Autodesk Fusion 360 part; units mm, degrees
(part 5 of 14)
  line L2140 (528.9162, 201.6125) -> (534.4154, 192.0875)
  line L2141 (534.4154, 192.0875) -> (545.4139, 192.0875)
  line L2142 (550.9132, 201.6125) -> (545.4139, 211.1375)
  line L2143 (545.4139, 192.0875) -> (550.9132, 201.6125)
  line L2144 (564.6614, 222.25) -> (553.6628, 222.25)
  line L2145 (553.6628, 222.25) -> (548.1636, 212.725)
  line L2146 (548.1636, 212.725) -> (553.6628, 203.2)
  line L2147 (553.6628, 203.2) -> (564.6614, 203.2)
  line L2148 (570.1606, 212.725) -> (564.6614, 222.25)
  line L2149 (564.6614, 203.2) -> (570.1606, 212.725)
  line L2150 (583.9088, 233.3625) -> (572.9102, 233.3625)
  line L2151 (572.9102, 233.3625) -> (567.411, 223.8375)
  line L2152 (567.411, 223.8375) -> (572.9102, 214.3125)
  line L2153 (572.9102, 214.3125) -> (583.9088, 214.3125)
  line L2154 (589.408, 223.8375) -> (583.9088, 233.3625)
  line L2155 (583.9088, 214.3125) -> (589.408, 223.8375)
  line L2156 (603.1562, 244.475) -> (592.1577, 244.475)
  line L2157 (592.1577, 244.475) -> (586.6584, 234.95)
  line L2158 (586.6584, 234.95) -> (592.1577, 225.425)
  line L2159 (592.1577, 225.425) -> (603.1562, 225.425)
  line L2160 (608.6554, 234.95) -> (603.1562, 244.475)
  line L2161 (603.1562, 225.425) -> (608.6554, 234.95)
  line L2162 (622.4036, 255.5875) -> (611.4051, 255.5875)
  line L2163 (611.4051, 255.5875) -> (605.9058, 246.0625)
  line L2164 (605.9058, 246.0625) -> (611.4051, 236.5375)
  line L2165 (611.4051, 236.5375) -> (622.4036, 236.5375)
  line L2166 (627.9029, 246.0625) -> (622.4036, 255.5875)
  line L2167 (622.4036, 236.5375) -> (627.9029, 246.0625)
  line L2168 (641.651, 266.7) -> (630.6525, 266.7)
  line L2169 (630.6525, 266.7) -> (625.1532, 257.175)
  line L2170 (625.1532, 257.175) -> (630.6525, 247.65)
  line L2171 (630.6525, 247.65) -> (641.651, 247.65)
  line L2172 (647.1503, 257.175) -> (641.651, 266.7)
  line L2173 (641.651, 247.65) -> (647.1503, 257.175)
  line L2174 (660.8984, 277.8125) -> (649.8999, 277.8125)
  line L2175 (649.8999, 277.8125) -> (644.4006, 268.2875)
  line L2176 (644.4006, 268.2875) -> (649.8999, 258.7625)
  line L2177 (649.8999, 258.7625) -> (660.8984, 258.7625)
  line L2178 (666.3977, 268.2875) -> (660.8984, 277.8125)
  line L2179 (660.8984, 258.7625) -> (666.3977, 268.2875)
  line L2180 (-493.9464, -366.7125) -> (-504.945, -366.7125)
  line L2181 (-504.945, -366.7125) -> (-510.4442, -376.2375)
  line L2182 (-510.4442, -376.2375) -> (-504.945, -385.7625)
  line L2183 (-504.945, -385.7625) -> (-493.9464, -385.7625)
  line L2184 (-488.4472, -376.2375) -> (-493.9464, -366.7125)
  line L2185 (-493.9464, -385.7625) -> (-488.4472, -376.2375)
  line L2186 (-474.699, -355.6) -> (-485.6976, -355.6)
  line L2187 (-485.6976, -355.6) -> (-491.1968, -365.125)
  line L2188 (-491.1968, -365.125) -> (-485.6976, -374.65)
  line L2189 (-485.6976, -374.65) -> (-474.699, -374.65)
  line L2190 (-469.1998, -365.125) -> (-474.699, -355.6)
  line L2191 (-474.699, -374.65) -> (-469.1998, -365.125)
  line L2192 (-455.4516, -344.4875) -> (-466.4501, -344.4875)
  line L2193 (-466.4501, -344.4875) -> (-471.9494, -354.0125)
  line L2194 (-471.9494, -354.0125) -> (-466.4501, -363.5375)
  line L2195 (-466.4501, -363.5375) -> (-455.4516, -363.5375)
  line L2196 (-449.9524, -354.0125) -> (-455.4516, -344.4875)
  line L2197 (-455.4516, -363.5375) -> (-449.9524, -354.0125)
  line L2198 (-436.2042, -333.375) -> (-447.2027, -333.375)
  line L2199 (-447.2027, -333.375) -> (-452.702, -342.9)
  line L2200 (-452.702, -342.9) -> (-447.2027, -352.425)
  line L2201 (-447.2027, -352.425) -> (-436.2042, -352.425)
  line L2202 (-430.7049, -342.9) -> (-436.2042, -333.375)
  line L2203 (-436.2042, -352.425) -> (-430.7049, -342.9)
  line L2204 (-416.9568, -322.2625) -> (-427.9553, -322.2625)
  line L2205 (-427.9553, -322.2625) -> (-433.4546, -331.7875)
  line L2206 (-433.4546, -331.7875) -> (-427.9553, -341.3125)
  line L2207 (-427.9553, -341.3125) -> (-416.9568, -341.3125)
  line L2208 (-411.4575, -331.7875) -> (-416.9568, -322.2625)
  line L2209 (-416.9568, -341.3125) -> (-411.4575, -331.7875)
  line L2210 (-397.7094, -311.15) -> (-408.7079, -311.15)
  line L2211 (-408.7079, -311.15) -> (-414.2072, -320.675)
  line L2212 (-414.2072, -320.675) -> (-408.7079, -330.2)
  line L2213 (-408.7079, -330.2) -> (-397.7094, -330.2)
  line L2214 (-392.2101, -320.675) -> (-397.7094, -311.15)
  line L2215 (-397.7094, -330.2) -> (-392.2101, -320.675)
  line L2216 (-378.462, -300.0375) -> (-389.4605, -300.0375)
  line L2217 (-389.4605, -300.0375) -> (-394.9597, -309.5625)
  line L2218 (-394.9597, -309.5625) -> (-389.4605, -319.0875)
  line L2219 (-389.4605, -319.0875) -> (-378.462, -319.0875)
  line L2220 (-372.9627, -309.5625) -> (-378.462, -300.0375)
  line L2221 (-378.462, -319.0875) -> (-372.9627, -309.5625)
  line L2222 (-359.2145, -288.925) -> (-370.2131, -288.925)
  line L2223 (-370.2131, -288.925) -> (-375.7123, -298.45)
  line L2224 (-375.7123, -298.45) -> (-370.2131, -307.975)
  line L2225 (-370.2131, -307.975) -> (-359.2145, -307.975)
  line L2226 (-353.7153, -298.45) -> (-359.2145, -288.925)
  line L2227 (-359.2145, -307.975) -> (-353.7153, -298.45)
  line L2228 (-339.9671, -277.8125) -> (-350.9657, -277.8125)
  line L2229 (-350.9657, -277.8125) -> (-356.4649, -287.3375)
  line L2230 (-356.4649, -287.3375) -> (-350.9657, -296.8625)
  line L2231 (-350.9657, -296.8625) -> (-339.9671, -296.8625)
  line L2232 (-334.4679, -287.3375) -> (-339.9671, -277.8125)
  line L2233 (-339.9671, -296.8625) -> (-334.4679, -287.3375)
  line L2234 (-320.7197, -266.7) -> (-331.7182, -266.7)
  line L2235 (-331.7182, -266.7) -> (-337.2175, -276.225)
  line L2236 (-337.2175, -276.225) -> (-331.7182, -285.75)
  line L2237 (-331.7182, -285.75) -> (-320.7197, -285.75)
  line L2238 (-315.2205, -276.225) -> (-320.7197, -266.7)
  line L2239 (-320.7197, -285.75) -> (-315.2205, -276.225)
  line L2240 (-301.4723, -255.5875) -> (-312.4708, -255.5875)
  line L2241 (-312.4708, -255.5875) -> (-317.9701, -265.1125)
  line L2242 (-317.9701, -265.1125) -> (-312.4708, -274.6375)
  line L2243 (-312.4708, -274.6375) -> (-301.4723, -274.6375)
  line L2244 (-295.973, -265.1125) -> (-301.4723, -255.5875)
  line L2245 (-301.4723, -274.6375) -> (-295.973, -265.1125)
  line L2246 (-282.2249, -244.475) -> (-293.2234, -244.475)
  line L2247 (-293.2234, -244.475) -> (-298.7227, -254)
  line L2248 (-298.7227, -254) -> (-293.2234, -263.525)
  line L2249 (-293.2234, -263.525) -> (-282.2249, -263.525)
  line L2250 (-276.7256, -254) -> (-282.2249, -244.475)
  line L2251 (-282.2249, -263.525) -> (-276.7256, -254)
  line L2252 (-262.9775, -233.3625) -> (-273.976, -233.3625)
  line L2253 (-273.976, -233.3625) -> (-279.4753, -242.8875)
  line L2254 (-279.4753, -242.8875) -> (-273.976, -252.4125)
  line L2255 (-273.976, -252.4125) -> (-262.9775, -252.4125)
  line L2256 (-257.4782, -242.8875) -> (-262.9775, -233.3625)
  line L2257 (-262.9775, -252.4125) -> (-257.4782, -242.8875)
  line L2258 (-243.7301, -222.25) -> (-254.7286, -222.25)
  line L2259 (-254.7286, -222.25) -> (-260.2278, -231.775)
  line L2260 (-260.2278, -231.775) -> (-254.7286, -241.3)
  line L2261 (-254.7286, -241.3) -> (-243.7301, -241.3)
  line L2262 (-238.2308, -231.775) -> (-243.7301, -222.25)
  line L2263 (-243.7301, -241.3) -> (-238.2308, -231.775)
  line L2264 (-224.4826, -211.1375) -> (-235.4812, -211.1375)
  line L2265 (-235.4812, -211.1375) -> (-240.9804, -220.6625)
  line L2266 (-240.9804, -220.6625) -> (-235.4812, -230.1875)
  line L2267 (-235.4812, -230.1875) -> (-224.4826, -230.1875)
  line L2268 (-218.9834, -220.6625) -> (-224.4826, -211.1375)
  line L2269 (-224.4826, -230.1875) -> (-218.9834, -220.6625)
  line L2270 (-205.2352, -200.025) -> (-216.2337, -200.025)
  line L2271 (-216.2337, -200.025) -> (-221.733, -209.55)
  line L2272 (-221.733, -209.55) -> (-216.2337, -219.075)
  line L2273 (-216.2337, -219.075) -> (-205.2352, -219.075)
  line L2274 (-199.736, -209.55) -> (-205.2352, -200.025)
  line L2275 (-205.2352, -219.075) -> (-199.736, -209.55)
  line L2276 (-185.9878, -188.9125) -> (-196.9863, -188.9125)
  line L2277 (-196.9863, -188.9125) -> (-202.4856, -198.4375)
  line L2278 (-202.4856, -198.4375) -> (-196.9863, -207.9625)
  line L2279 (-196.9863, -207.9625) -> (-185.9878, -207.9625)
  line L2280 (-180.4886, -198.4375) -> (-185.9878, -188.9125)
  line L2281 (-185.9878, -207.9625) -> (-180.4886, -198.4375)
  line L2282 (-166.7404, -177.8) -> (-177.7389, -177.8)
  line L2283 (-177.7389, -177.8) -> (-183.2382, -187.325)
  line L2284 (-183.2382, -187.325) -> (-177.7389, -196.85)
  line L2285 (-177.7389, -196.85) -> (-166.7404, -196.85)
  line L2286 (-161.2411, -187.325) -> (-166.7404, -177.8)
  line L2287 (-166.7404, -196.85) -> (-161.2411, -187.325)
  line L2288 (-147.493, -166.6875) -> (-158.4915, -166.6875)
  line L2289 (-158.4915, -166.6875) -> (-163.9908, -176.2125)
  line L2290 (-163.9908, -176.2125) -> (-158.4915, -185.7375)
  line L2291 (-158.4915, -185.7375) -> (-147.493, -185.7375)
  line L2292 (-141.9937, -176.2125) -> (-147.493, -166.6875)
  line L2293 (-147.493, -185.7375) -> (-141.9937, -176.2125)
  line L2294 (-128.2456, -155.575) -> (-139.2441, -155.575)
  line L2295 (-139.2441, -155.575) -> (-144.7434, -165.1)
  line L2296 (-144.7434, -165.1) -> (-139.2441, -174.625)
  line L2297 (-139.2441, -174.625) -> (-128.2456, -174.625)
  line L2298 (-122.7463, -165.1) -> (-128.2456, -155.575)
  line L2299 (-128.2456, -174.625) -> (-122.7463, -165.1)
  line L2300 (-108.9982, -144.4625) -> (-119.9967, -144.4625)
  line L2301 (-119.9967, -144.4625) -> (-125.4959, -153.9875)
  line L2302 (-125.4959, -153.9875) -> (-119.9967, -163.5125)
  line L2303 (-119.9967, -163.5125) -> (-108.9982, -163.5125)
  line L2304 (-103.4989, -153.9875) -> (-108.9982, -144.4625)
  line L2305 (-108.9982, -163.5125) -> (-103.4989, -153.9875)
  line L2306 (-89.7507, -133.35) -> (-100.7493, -133.35)
  line L2307 (-100.7493, -133.35) -> (-106.2485, -142.875)
  line L2308 (-106.2485, -142.875) -> (-100.7493, -152.4)
  line L2309 (-100.7493, -152.4) -> (-89.7507, -152.4)
  line L2310 (-84.2515, -142.875) -> (-89.7507, -133.35)
  line L2311 (-89.7507, -152.4) -> (-84.2515, -142.875)
  line L2312 (-70.5033, -122.2375) -> (-81.5018, -122.2375)
  line L2313 (-81.5018, -122.2375) -> (-87.0011, -131.7625)
  line L2314 (-87.0011, -131.7625) -> (-81.5018, -141.2875)
  line L2315 (-81.5018, -141.2875) -> (-70.5033, -141.2875)
  line L2316 (-65.0041, -131.7625) -> (-70.5033, -122.2375)
  line L2317 (-70.5033, -141.2875) -> (-65.0041, -131.7625)
  line L2318 (-51.2559, -111.125) -> (-62.2544, -111.125)
  line L2319 (-62.2544, -111.125) -> (-67.7537, -120.65)
  line L2320 (-67.7537, -120.65) -> (-62.2544, -130.175)
  line L2321 (-62.2544, -130.175) -> (-51.2559, -130.175)
  line L2322 (-45.7566, -120.65) -> (-51.2559, -111.125)
  line L2323 (-51.2559, -130.175) -> (-45.7566, -120.65)
  line L2324 (-32.0085, -100.0125) -> (-43.007, -100.0125)
  line L2325 (-43.007, -100.0125) -> (-48.5063, -109.5375)
  line L2326 (-48.5063, -109.5375) -> (-43.007, -119.0625)
  line L2327 (-43.007, -119.0625) -> (-32.0085, -119.0625)
  line L2328 (-26.5092, -109.5375) -> (-32.0085, -100.0125)
  line L2329 (-32.0085, -119.0625) -> (-26.5092, -109.5375)
  line L2330 (-12.7611, -88.9) -> (-23.7596, -88.9)
  line L2331 (-23.7596, -88.9) -> (-29.2589, -98.425)
  line L2332 (-29.2589, -98.425) -> (-23.7596, -107.95)
  line L2333 (-23.7596, -107.95) -> (-12.7611, -107.95)
  line L2334 (-7.2618, -98.425) -> (-12.7611, -88.9)
  line L2335 (-12.7611, -107.95) -> (-7.2618, -98.425)
  line L2336 (6.4863, -77.7875) -> (-4.5122, -77.7875)
  line L2337 (-4.5122, -77.7875) -> (-10.0114, -87.3125)
  line L2338 (-10.0114, -87.3125) -> (-4.5122, -96.8375)
  line L2339 (-4.5122, -96.8375) -> (6.4863, -96.8375)
  line L2340 (11.9856, -87.3125) -> (6.4863, -77.7875)
  line L2341 (6.4863, -96.8375) -> (11.9856, -87.3125)
  line L2342 (25.7337, -66.675) -> (14.7352, -66.675)
  line L2343 (14.7352, -66.675) -> (9.236, -76.2)
  line L2344 (9.236, -76.2) -> (14.7352, -85.725)
  line L2345 (14.7352, -85.725) -> (25.7337, -85.725)
  line L2346 (31.233, -76.2) -> (25.7337, -66.675)
  line L2347 (25.7337, -85.725) -> (31.233, -76.2)
  line L2348 (44.9812, -55.5625) -> (33.9826, -55.5625)
  line L2349 (33.9826, -55.5625) -> (28.4834, -65.0875)
  line L2350 (28.4834, -65.0875) -> (33.9826, -74.6125)
  line L2351 (33.9826, -74.6125) -> (44.9812, -74.6125)
  line L2352 (50.4804, -65.0875) -> (44.9812, -55.5625)
  line L2353 (44.9812, -74.6125) -> (50.4804, -65.0875)
  line L2354 (64.2286, -44.45) -> (53.2301, -44.45)
  line L2355 (53.2301, -44.45) -> (47.7308, -53.975)
  line L2356 (47.7308, -53.975) -> (53.2301, -63.5)
  line L2357 (53.2301, -63.5) -> (64.2286, -63.5)
  line L2358 (69.7278, -53.975) -> (64.2286, -44.45)
  line L2359 (64.2286, -63.5) -> (69.7278, -53.975)
  line L2360 (83.476, -33.3375) -> (72.4775, -33.3375)
  line L2361 (72.4775, -33.3375) -> (66.9782, -42.8625)
  line L2362 (66.9782, -42.8625) -> (72.4775, -52.3875)
  line L2363 (72.4775, -52.3875) -> (83.476, -52.3875)
  line L2364 (88.9753, -42.8625) -> (83.476, -33.3375)
  line L2365 (83.476, -52.3875) -> (88.9753, -42.8625)
  line L2366 (102.7234, -22.225) -> (91.7249, -22.225)
  line L2367 (91.7249, -22.225) -> (86.2256, -31.75)
  line L2368 (86.2256, -31.75) -> (91.7249, -41.275)
  line L2369 (91.7249, -41.275) -> (102.7234, -41.275)
  line L2370 (108.2227, -31.75) -> (102.7234, -22.225)
  line L2371 (102.7234, -41.275) -> (108.2227, -31.75)
  line L2372 (121.9708, -11.1125) -> (110.9723, -11.1125)
  line L2373 (110.9723, -11.1125) -> (105.473, -20.6375)
  line L2374 (105.473, -20.6375) -> (110.9723, -30.1625)
  line L2375 (110.9723, -30.1625) -> (121.9708, -30.1625)
  line L2376 (127.4701, -20.6375) -> (121.9708, -11.1125)
  line L2377 (121.9708, -30.1625) -> (127.4701, -20.6375)
  line L2378 (141.2182, 0) -> (130.2197, 0)
  line L2379 (130.2197, 0) -> (124.7205, -9.525)
  line L2380 (124.7205, -9.525) -> (130.2197, -19.05)
  line L2381 (130.2197, -19.05) -> (141.2182, -19.05)
  line L2382 (146.7175, -9.525) -> (141.2182, 0)
  line L2383 (141.2182, -19.05) -> (146.7175, -9.525)
  line L2384 (160.4657, 11.1125) -> (149.4671, 11.1125)
  line L2385 (149.4671, 11.1125) -> (143.9679, 1.5875)
  line L2386 (143.9679, 1.5875) -> (149.4671, -7.9375)
  line L2387 (149.4671, -7.9375) -> (160.4657, -7.9375)
  line L2388 (165.9649, 1.5875) -> (160.4657, 11.1125)
  line L2389 (160.4657, -7.9375) -> (165.9649, 1.5875)
  line L2390 (179.7131, 22.225) -> (168.7145, 22.225)
  line L2391 (168.7145, 22.225) -> (163.2153, 12.7)
  line L2392 (163.2153, 12.7) -> (168.7145, 3.175)
  line L2393 (168.7145, 3.175) -> (179.7131, 3.175)
  line L2394 (185.2123, 12.7) -> (179.7131, 22.225)
  line L2395 (179.7131, 3.175) -> (185.2123, 12.7)
  line L2396 (198.9605, 33.3375) -> (187.962, 33.3375)
  line L2397 (187.962, 33.3375) -> (182.4627, 23.8125)
  line L2398 (182.4627, 23.8125) -> (187.962, 14.2875)
  line L2399 (187.962, 14.2875) -> (198.9605, 14.2875)
  line L2400 (204.4597, 23.8125) -> (198.9605, 33.3375)
  line L2401 (198.9605, 14.2875) -> (204.4597, 23.8125)
  line L2402 (218.2079, 44.45) -> (207.2094, 44.45)
  line L2403 (207.2094, 44.45) -> (201.7101, 34.925)
  line L2404 (201.7101, 34.925) -> (207.2094, 25.4)
  line L2405 (207.2094, 25.4) -> (218.2079, 25.4)
  line L2406 (223.7072, 34.925) -> (218.2079, 44.45)
  line L2407 (218.2079, 25.4) -> (223.7072, 34.925)
  line L2408 (237.4553, 55.5625) -> (226.4568, 55.5625)
  line L2409 (226.4568, 55.5625) -> (220.9575, 46.0375)
  line L2410 (220.9575, 46.0375) -> (226.4568, 36.5125)
  line L2411 (226.4568, 36.5125) -> (237.4553, 36.5125)
  line L2412 (242.9546, 46.0375) -> (237.4553, 55.5625)
  line L2413 (237.4553, 36.5125) -> (242.9546, 46.0375)
  line L2414 (256.7027, 66.675) -> (245.7042, 66.675)
  line L2415 (245.7042, 66.675) -> (240.2049, 57.15)
  line L2416 (240.2049, 57.15) -> (245.7042, 47.625)
  line L2417 (245.7042, 47.625) -> (256.7027, 47.625)
  line L2418 (262.202, 57.15) -> (256.7027, 66.675)
  line L2419 (256.7027, 47.625) -> (262.202, 57.15)
  line L2420 (275.9501, 77.7875) -> (264.9516, 77.7875)
  line L2421 (264.9516, 77.7875) -> (259.4524, 68.2625)
  line L2422 (259.4524, 68.2625) -> (264.9516, 58.7375)
  line L2423 (264.9516, 58.7375) -> (275.9501, 58.7375)
  line L2424 (281.4494, 68.2625) -> (275.9501, 77.7875)
  line L2425 (275.9501, 58.7375) -> (281.4494, 68.2625)
  line L2426 (295.1976, 88.9) -> (284.199, 88.9)
  line L2427 (284.199, 88.9) -> (278.6998, 79.375)
  line L2428 (278.6998, 79.375) -> (284.199, 69.85)
  line L2429 (284.199, 69.85) -> (295.1976, 69.85)
  line L2430 (300.6968, 79.375) -> (295.1976, 88.9)
  line L2431 (295.1976, 69.85) -> (300.6968, 79.375)
  line L2432 (314.445, 100.0125) -> (303.4464, 100.0125)
  line L2433 (303.4464, 100.0125) -> (297.9472, 90.4875)
  line L2434 (297.9472, 90.4875) -> (303.4464, 80.9625)
  line L2435 (303.4464, 80.9625) -> (314.445, 80.9625)
  line L2436 (319.9442, 90.4875) -> (314.445, 100.0125)
  line L2437 (314.445, 80.9625) -> (319.9442, 90.4875)
  line L2438 (333.6924, 111.125) -> (322.6939, 111.125)
  line L2439 (322.6939, 111.125) -> (317.1946, 101.6)
  line L2440 (317.1946, 101.6) -> (322.6939, 92.075)
  line L2441 (322.6939, 92.075) -> (333.6924, 92.075)
  line L2442 (339.1916, 101.6) -> (333.6924, 111.125)
  line L2443 (333.6924, 92.075) -> (339.1916, 101.6)
  line L2444 (352.9398, 122.2375) -> (341.9413, 122.2375)
  line L2445 (341.9413, 122.2375) -> (336.442, 112.7125)
  line L2446 (336.442, 112.7125) -> (341.9413, 103.1875)
  line L2447 (341.9413, 103.1875) -> (352.9398, 103.1875)
  line L2448 (358.4391, 112.7125) -> (352.9398, 122.2375)
  line L2449 (352.9398, 103.1875) -> (358.4391, 112.7125)
  line L2450 (372.1872, 133.35) -> (361.1887, 133.35)
  line L2451 (361.1887, 133.35) -> (355.6894, 123.825)
  line L2452 (355.6894, 123.825) -> (361.1887, 114.3)
  line L2453 (361.1887, 114.3) -> (372.1872, 114.3)
  line L2454 (377.6865, 123.825) -> (372.1872, 133.35)
  line L2455 (372.1872, 114.3) -> (377.6865, 123.825)
  line L2456 (391.4346, 144.4625) -> (380.4361, 144.4625)
  line L2457 (380.4361, 144.4625) -> (374.9368, 134.9375)
  line L2458 (374.9368, 134.9375) -> (380.4361, 125.4125)
  line L2459 (380.4361, 125.4125) -> (391.4346, 125.4125)
  line L2460 (396.9339, 134.9375) -> (391.4346, 144.4625)
  line L2461 (391.4346, 125.4125) -> (396.9339, 134.9375)
  line L2462 (410.682, 155.575) -> (399.6835, 155.575)
  line L2463 (399.6835, 155.575) -> (394.1843, 146.05)
  line L2464 (394.1843, 146.05) -> (399.6835, 136.525)
  line L2465 (399.6835, 136.525) -> (410.682, 136.525)
  line L2466 (416.1813, 146.05) -> (410.682, 155.575)
  line L2467 (410.682, 136.525) -> (416.1813, 146.05)
  line L2468 (429.9295, 166.6875) -> (418.9309, 166.6875)
  line L2469 (418.9309, 166.6875) -> (413.4317, 157.1625)
  line L2470 (413.4317, 157.1625) -> (418.9309, 147.6375)
  line L2471 (418.9309, 147.6375) -> (429.9295, 147.6375)
  line L2472 (435.4287, 157.1625) -> (429.9295, 166.6875)
  line L2473 (429.9295, 147.6375) -> (435.4287, 157.1625)
  line L2474 (449.1769, 177.8) -> (438.1783, 177.8)
  line L2475 (438.1783, 177.8) -> (432.6791, 168.275)
  line L2476 (432.6791, 168.275) -> (438.1783, 158.75)
  line L2477 (438.1783, 158.75) -> (449.1769, 158.75)
  line L2478 (454.6761, 168.275) -> (449.1769, 177.8)
  line L2479 (449.1769, 158.75) -> (454.6761, 168.275)
  line L2480 (468.4243, 188.9125) -> (457.4258, 188.9125)
  line L2481 (457.4258, 188.9125) -> (451.9265, 179.3875)
  line L2482 (451.9265, 179.3875) -> (457.4258, 169.8625)
  line L2483 (457.4258, 169.8625) -> (468.4243, 169.8625)
  line L2484 (473.9235, 179.3875) -> (468.4243, 188.9125)
  line L2485 (468.4243, 169.8625) -> (473.9235, 179.3875)
  line L2486 (487.6717, 200.025) -> (476.6732, 200.025)
  line L2487 (476.6732, 200.025) -> (471.1739, 190.5)
  line L2488 (471.1739, 190.5) -> (476.6732, 180.975)
  line L2489 (476.6732, 180.975) -> (487.6717, 180.975)
  line L2490 (493.171, 190.5) -> (487.6717, 200.025)
  line L2491 (487.6717, 180.975) -> (493.171, 190.5)
  line L2492 (506.9191, 211.1375) -> (495.9206, 211.1375)
  line L2493 (495.9206, 211.1375) -> (490.4213, 201.6125)
  line L2494 (490.4213, 201.6125) -> (495.9206, 192.0875)
  line L2495 (495.9206, 192.0875) -> (506.9191, 192.0875)
  line L2496 (512.4184, 201.6125) -> (506.9191, 211.1375)
  line L2497 (506.9191, 192.0875) -> (512.4184, 201.6125)
  line L2498 (526.1665, 222.25) -> (515.168, 222.25)
  line L2499 (515.168, 222.25) -> (509.6687, 212.725)
  line L2500 (509.6687, 212.725) -> (515.168, 203.2)
  line L2501 (515.168, 203.2) -> (526.1665, 203.2)
  line L2502 (531.6658, 212.725) -> (526.1665, 222.25)
  line L2503 (526.1665, 203.2) -> (531.6658, 212.725)
  line L2504 (545.4139, 233.3625) -> (534.4154, 233.3625)
  line L2505 (534.4154, 233.3625) -> (528.9162, 223.8375)
  line L2506 (528.9162, 223.8375) -> (534.4154, 214.3125)
  line L2507 (534.4154, 214.3125) -> (545.4139, 214.3125)
  line L2508 (550.9132, 223.8375) -> (545.4139, 233.3625)
  line L2509 (545.4139, 214.3125) -> (550.9132, 223.8375)
  line L2510 (564.6614, 244.475) -> (553.6628, 244.475)
  line L2511 (553.6628, 244.475) -> (548.1636, 234.95)
  line L2512 (548.1636, 234.95) -> (553.6628, 225.425)
  line L2513 (553.6628, 225.425) -> (564.6614, 225.425)
  line L2514 (570.1606, 234.95) -> (564.6614, 244.475)
  line L2515 (564.6614, 225.425) -> (570.1606, 234.95)
  line L2516 (583.9088, 255.5875) -> (572.9102, 255.5875)
  line L2517 (572.9102, 255.5875) -> (567.411, 246.0625)
  line L2518 (567.411, 246.0625) -> (572.9102, 236.5375)
  line L2519 (572.9102, 236.5375) -> (583.9088, 236.5375)
  line L2520 (589.408, 246.0625) -> (583.9088, 255.5875)
  line L2521 (583.9088, 236.5375) -> (589.408, 246.0625)
  line L2522 (603.1562, 266.7) -> (592.1577, 266.7)
  line L2523 (592.1577, 266.7) -> (586.6584, 257.175)
  line L2524 (586.6584, 257.175) -> (592.1577, 247.65)
  line L2525 (592.1577, 247.65) -> (603.1562, 247.65)
  line L2526 (608.6554, 257.175) -> (603.1562, 266.7)
  line L2527 (603.1562, 247.65) -> (608.6554, 257.175)
  line L2528 (622.4036, 277.8125) -> (611.4051, 277.8125)
  line L2529 (611.4051, 277.8125) -> (605.9058, 268.2875)
  line L2530 (605.9058, 268.2875) -> (611.4051, 258.7625)
  line L2531 (611.4051, 258.7625) -> (622.4036, 258.7625)
  line L2532 (627.9029, 268.2875) -> (622.4036, 277.8125)
  line L2533 (622.4036, 258.7625) -> (627.9029, 268.2875)
  line L2534 (641.651, 288.925) -> (630.6525, 288.925)
  line L2535 (630.6525, 288.925) -> (625.1532, 279.4)
  line L2536 (625.1532, 279.4) -> (630.6525, 269.875)
  line L2537 (630.6525, 269.875) -> (641.651, 269.875)
  line L2538 (647.1503, 279.4) -> (641.651, 288.925)
  line L2539 (641.651, 269.875) -> (647.1503, 279.4)
  line L2540 (-513.1939, -355.6) -> (-524.1924, -355.6)
  line L2541 (-524.1924, -355.6) -> (-529.6916, -365.125)
  line L2542 (-529.6916, -365.125) -> (-524.1924, -374.65)
  line L2543 (-524.1924, -374.65) -> (-513.1939, -374.65)
  line L2544 (-507.6946, -365.125) -> (-513.1939, -355.6)
  line L2545 (-513.1939, -374.65) -> (-507.6946, -365.125)
  line L2546 (-493.9464, -344.4875) -> (-504.945, -344.4875)
  line L2547 (-504.945, -344.4875) -> (-510.4442, -354.0125)
  line L2548 (-510.4442, -354.0125) -> (-504.945, -363.5375)
  line L2549 (-504.945, -363.5375) -> (-493.9464, -363.5375)
  line L2550 (-488.4472, -354.0125) -> (-493.9464, -344.4875)
  line L2551 (-493.9464, -363.5375) -> (-488.4472, -354.0125)
  line L2552 (-474.699, -333.375) -> (-485.6976, -333.375)
  line L2553 (-485.6976, -333.375) -> (-491.1968, -342.9)
  line L2554 (-491.1968, -342.9) -> (-485.6976, -352.425)
  line L2555 (-485.6976, -352.425) -> (-474.699, -352.425)
  line L2556 (-469.1998, -342.9) -> (-474.699, -333.375)
  line L2557 (-474.699, -352.425) -> (-469.1998, -342.9)
  line L2558 (-455.4516, -322.2625) -> (-466.4501, -322.2625)
  line L2559 (-466.4501, -322.2625) -> (-471.9494, -331.7875)
  line L2560 (-471.9494, -331.7875) -> (-466.4501, -341.3125)
  line L2561 (-466.4501, -341.3125) -> (-455.4516, -341.3125)
  line L2562 (-449.9524, -331.7875) -> (-455.4516, -322.2625)
  line L2563 (-455.4516, -341.3125) -> (-449.9524, -331.7875)
  line L2564 (-436.2042, -311.15) -> (-447.2027, -311.15)
  line L2565 (-447.2027, -311.15) -> (-452.702, -320.675)
  line L2566 (-452.702, -320.675) -> (-447.2027, -330.2)
  line L2567 (-447.2027, -330.2) -> (-436.2042, -330.2)
  line L2568 (-430.7049, -320.675) -> (-436.2042, -311.15)
  line L2569 (-436.2042, -330.2) -> (-430.7049, -320.675)
  line L2570 (-416.9568, -300.0375) -> (-427.9553, -300.0375)
  line L2571 (-427.9553, -300.0375) -> (-433.4546, -309.5625)
  line L2572 (-433.4546, -309.5625) -> (-427.9553, -319.0875)
  line L2573 (-427.9553, -319.0875) -> (-416.9568, -319.0875)
  line L2574 (-411.4575, -309.5625) -> (-416.9568, -300.0375)
  line L2575 (-416.9568, -319.0875) -> (-411.4575, -309.5625)
  line L2576 (-397.7094, -288.925) -> (-408.7079, -288.925)
  line L2577 (-408.7079, -288.925) -> (-414.2072, -298.45)
  line L2578 (-414.2072, -298.45) -> (-408.7079, -307.975)
  line L2579 (-408.7079, -307.975) -> (-397.7094, -307.975)
  line L2580 (-392.2101, -298.45) -> (-397.7094, -288.925)
  line L2581 (-397.7094, -307.975) -> (-392.2101, -298.45)
  line L2582 (-378.462, -277.8125) -> (-389.4605, -277.8125)
  line L2583 (-389.4605, -277.8125) -> (-394.9597, -287.3375)
  line L2584 (-394.9597, -287.3375) -> (-389.4605, -296.8625)
  line L2585 (-389.4605, -296.8625) -> (-378.462, -296.8625)
  line L2586 (-372.9627, -287.3375) -> (-378.462, -277.8125)
  line L2587 (-378.462, -296.8625) -> (-372.9627, -287.3375)
  line L2588 (-359.2145, -266.7) -> (-370.2131, -266.7)
  line L2589 (-370.2131, -266.7) -> (-375.7123, -276.225)
  line L2590 (-375.7123, -276.225) -> (-370.2131, -285.75)
  line L2591 (-370.2131, -285.75) -> (-359.2145, -285.75)
  line L2592 (-353.7153, -276.225) -> (-359.2145, -266.7)
  line L2593 (-359.2145, -285.75) -> (-353.7153, -276.225)
  line L2594 (-339.9671, -255.5875) -> (-350.9657, -255.5875)
  line L2595 (-350.9657, -255.5875) -> (-356.4649, -265.1125)
  line L2596 (-356.4649, -265.1125) -> (-350.9657, -274.6375)
  line L2597 (-350.9657, -274.6375) -> (-339.9671, -274.6375)
  line L2598 (-334.4679, -265.1125) -> (-339.9671, -255.5875)
  line L2599 (-339.9671, -274.6375) -> (-334.4679, -265.1125)
  line L2600 (-320.7197, -244.475) -> (-331.7182, -244.475)
  line L2601 (-331.7182, -244.475) -> (-337.2175, -254)
  line L2602 (-337.2175, -254) -> (-331.7182, -263.525)
  line L2603 (-331.7182, -263.525) -> (-320.7197, -263.525)
  line L2604 (-315.2205, -254) -> (-320.7197, -244.475)
  line L2605 (-320.7197, -263.525) -> (-315.2205, -254)
  line L2606 (-301.4723, -233.3625) -> (-312.4708, -233.3625)
  line L2607 (-312.4708, -233.3625) -> (-317.9701, -242.8875)
  line L2608 (-317.9701, -242.8875) -> (-312.4708, -252.4125)
  line L2609 (-312.4708, -252.4125) -> (-301.4723, -252.4125)
  line L2610 (-295.973, -242.8875) -> (-301.4723, -233.3625)
  line L2611 (-301.4723, -252.4125) -> (-295.973, -242.8875)
  line L2612 (-282.2249, -222.25) -> (-293.2234, -222.25)
  line L2613 (-293.2234, -222.25) -> (-298.7227, -231.775)
  line L2614 (-298.7227, -231.775) -> (-293.2234, -241.3)
  line L2615 (-293.2234, -241.3) -> (-282.2249, -241.3)
  line L2616 (-276.7256, -231.775) -> (-282.2249, -222.25)
  line L2617 (-282.2249, -241.3) -> (-276.7256, -231.775)
  line L2618 (-262.9775, -211.1375) -> (-273.976, -211.1375)
  line L2619 (-273.976, -211.1375) -> (-279.4753, -220.6625)
  line L2620 (-279.4753, -220.6625) -> (-273.976, -230.1875)
  line L2621 (-273.976, -230.1875) -> (-262.9775, -230.1875)
  line L2622 (-257.4782, -220.6625) -> (-262.9775, -211.1375)
  line L2623 (-262.9775, -230.1875) -> (-257.4782, -220.6625)
  line L2624 (-243.7301, -200.025) -> (-254.7286, -200.025)
  line L2625 (-254.7286, -200.025) -> (-260.2278, -209.55)
  line L2626 (-260.2278, -209.55) -> (-254.7286, -219.075)
  line L2627 (-254.7286, -219.075) -> (-243.7301, -219.075)
  line L2628 (-238.2308, -209.55) -> (-243.7301, -200.025)
  line L2629 (-243.7301, -219.075) -> (-238.2308, -209.55)
  line L2630 (-224.4826, -188.9125) -> (-235.4812, -188.9125)
  line L2631 (-235.4812, -188.9125) -> (-240.9804, -198.4375)
  line L2632 (-240.9804, -198.4375) -> (-235.4812, -207.9625)
  line L2633 (-235.4812, -207.9625) -> (-224.4826, -207.9625)
  line L2634 (-218.9834, -198.4375) -> (-224.4826, -188.9125)
  line L2635 (-224.4826, -207.9625) -> (-218.9834, -198.4375)
  line L2636 (-205.2352, -177.8) -> (-216.2337, -177.8)
  line L2637 (-216.2337, -177.8) -> (-221.733, -187.325)
  line L2638 (-221.733, -187.325) -> (-216.2337, -196.85)
  line L2639 (-216.2337, -196.85) -> (-205.2352, -196.85)
  line L2640 (-199.736, -187.325) -> (-205.2352, -177.8)
  line L2641 (-205.2352, -196.85) -> (-199.736, -187.325)
  line L2642 (-185.9878, -166.6875) -> (-196.9863, -166.6875)
  line L2643 (-196.9863, -166.6875) -> (-202.4856, -176.2125)
  line L2644 (-202.4856, -176.2125) -> (-196.9863, -185.7375)
  line L2645 (-196.9863, -185.7375) -> (-185.9878, -185.7375)
  line L2646 (-180.4886, -176.2125) -> (-185.9878, -166.6875)
  line L2647 (-185.9878, -185.7375) -> (-180.4886, -176.2125)
  line L2648 (-166.7404, -155.575) -> (-177.7389, -155.575)
  line L2649 (-177.7389, -155.575) -> (-183.2382, -165.1)
  line L2650 (-183.2382, -165.1) -> (-177.7389, -174.625)
  line L2651 (-177.7389, -174.625) -> (-166.7404, -174.625)
  line L2652 (-161.2411, -165.1) -> (-166.7404, -155.575)
  line L2653 (-166.7404, -174.625) -> (-161.2411, -165.1)
  line L2654 (-147.493, -144.4625) -> (-158.4915, -144.4625)
  line L2655 (-158.4915, -144.4625) -> (-163.9908, -153.9875)
  line L2656 (-163.9908, -153.9875) -> (-158.4915, -163.5125)
  line L2657 (-158.4915, -163.5125) -> (-147.493, -163.5125)
  line L2658 (-141.9937, -153.9875) -> (-147.493, -144.4625)
  line L2659 (-147.493, -163.5125) -> (-141.9937, -153.9875)
  line L2660 (-128.2456, -133.35) -> (-139.2441, -133.35)
  line L2661 (-139.2441, -133.35) -> (-144.7434, -142.875)
  line L2662 (-144.7434, -142.875) -> (-139.2441, -152.4)
  line L2663 (-139.2441, -152.4) -> (-128.2456, -152.4)
  line L2664 (-122.7463, -142.875) -> (-128.2456, -133.35)
  line L2665 (-128.2456, -152.4) -> (-122.7463, -142.875)
  line L2666 (-108.9982, -122.2375) -> (-119.9967, -122.2375)
  line L2667 (-119.9967, -122.2375) -> (-125.4959, -131.7625)
  line L2668 (-125.4959, -131.7625) -> (-119.9967, -141.2875)
  line L2669 (-119.9967, -141.2875) -> (-108.9982, -141.2875)
  line L2670 (-103.4989, -131.7625) -> (-108.9982, -122.2375)
  line L2671 (-108.9982, -141.2875) -> (-103.4989, -131.7625)
  line L2672 (-89.7507, -111.125) -> (-100.7493, -111.125)
  line L2673 (-100.7493, -111.125) -> (-106.2485, -120.65)
  line L2674 (-106.2485, -120.65) -> (-100.7493, -130.175)
  line L2675 (-100.7493, -130.175) -> (-89.7507, -130.175)
  line L2676 (-84.2515, -120.65) -> (-89.7507, -111.125)
  line L2677 (-89.7507, -130.175) -> (-84.2515, -120.65)
  line L2678 (-70.5033, -100.0125) -> (-81.5018, -100.0125)
  line L2679 (-81.5018, -100.0125) -> (-87.0011, -109.5375)
  line L2680 (-87.0011, -109.5375) -> (-81.5018, -119.0625)
  line L2681 (-81.5018, -119.0625) -> (-70.5033, -119.0625)
  line L2682 (-65.0041, -109.5375) -> (-70.5033, -100.0125)
  line L2683 (-70.5033, -119.0625) -> (-65.0041, -109.5375)
  line L2684 (-51.2559, -88.9) -> (-62.2544, -88.9)
  line L2685 (-62.2544, -88.9) -> (-67.7537, -98.425)
  line L2686 (-67.7537, -98.425) -> (-62.2544, -107.95)
  line L2687 (-62.2544, -107.95) -> (-51.2559, -107.95)
  line L2688 (-45.7566, -98.425) -> (-51.2559, -88.9)
  line L2689 (-51.2559, -107.95) -> (-45.7566, -98.425)
  line L2690 (-32.0085, -77.7875) -> (-43.007, -77.7875)
  line L2691 (-43.007, -77.7875) -> (-48.5063, -87.3125)
  line L2692 (-48.5063, -87.3125) -> (-43.007, -96.8375)
  line L2693 (-43.007, -96.8375) -> (-32.0085, -96.8375)
  line L2694 (-26.5092, -87.3125) -> (-32.0085, -77.7875)
  line L2695 (-32.0085, -96.8375) -> (-26.5092, -87.3125)
  line L2696 (-12.7611, -66.675) -> (-23.7596, -66.675)
  line L2697 (-23.7596, -66.675) -> (-29.2589, -76.2)
  line L2698 (-29.2589, -76.2) -> (-23.7596, -85.725)
  line L2699 (-23.7596, -85.725) -> (-12.7611, -85.725)
  line L2700 (-7.2618, -76.2) -> (-12.7611, -66.675)
  line L2701 (-12.7611, -85.725) -> (-7.2618, -76.2)
  line L2702 (6.4863, -55.5625) -> (-4.5122, -55.5625)
  line L2703 (-4.5122, -55.5625) -> (-10.0114, -65.0875)
  line L2704 (-10.0114, -65.0875) -> (-4.5122, -74.6125)
  line L2705 (-4.5122, -74.6125) -> (6.4863, -74.6125)
  line L2706 (11.9856, -65.0875) -> (6.4863, -55.5625)
  line L2707 (6.4863, -74.6125) -> (11.9856, -65.0875)
  line L2708 (25.7337, -44.45) -> (14.7352, -44.45)
  line L2709 (14.7352, -44.45) -> (9.236, -53.975)
  line L2710 (9.236, -53.975) -> (14.7352, -63.5)
  line L2711 (14.7352, -63.5) -> (25.7337, -63.5)
  line L2712 (31.233, -53.975) -> (25.7337, -44.45)
  line L2713 (25.7337, -63.5) -> (31.233, -53.975)
  line L2714 (44.9812, -33.3375) -> (33.9826, -33.3375)
  line L2715 (33.9826, -33.3375) -> (28.4834, -42.8625)
  line L2716 (28.4834, -42.8625) -> (33.9826, -52.3875)
  line L2717 (33.9826, -52.3875) -> (44.9812, -52.3875)
  line L2718 (50.4804, -42.8625) -> (44.9812, -33.3375)
  line L2719 (44.9812, -52.3875) -> (50.4804, -42.8625)
  line L2720 (64.2286, -22.225) -> (53.2301, -22.225)
  line L2721 (53.2301, -22.225) -> (47.7308, -31.75)
  line L2722 (47.7308, -31.75) -> (53.2301, -41.275)
  line L2723 (53.2301, -41.275) -> (64.2286, -41.275)
  line L2724 (69.7278, -31.75) -> (64.2286, -22.225)
  line L2725 (64.2286, -41.275) -> (69.7278, -31.75)
  line L2726 (83.476, -11.1125) -> (72.4775, -11.1125)
  line L2727 (72.4775, -11.1125) -> (66.9782, -20.6375)
  line L2728 (66.9782, -20.6375) -> (72.4775, -30.1625)
  line L2729 (72.4775, -30.1625) -> (83.476, -30.1625)
  line L2730 (88.9753, -20.6375) -> (83.476, -11.1125)
  line L2731 (83.476, -30.1625) -> (88.9753, -20.6375)
  line L2732 (102.7234, 0) -> (91.7249, 0)
  line L2733 (91.7249, 0) -> (86.2256, -9.525)
  line L2734 (86.2256, -9.525) -> (91.7249, -19.05)
  line L2735 (91.7249, -19.05) -> (102.7234, -19.05)
  line L2736 (108.2227, -9.525) -> (102.7234, 0)
  line L2737 (102.7234, -19.05) -> (108.2227, -9.525)
  line L2738 (121.9708, 11.1125) -> (110.9723, 11.1125)
  line L2739 (110.9723, 11.1125) -> (105.473, 1.5875)
  line L2740 (105.473, 1.5875) -> (110.9723, -7.9375)
  line L2741 (110.9723, -7.9375) -> (121.9708, -7.9375)
  line L2742 (127.4701, 1.5875) -> (121.9708, 11.1125)
  line L2743 (121.9708, -7.9375) -> (127.4701, 1.5875)
  line L2744 (141.2182, 22.225) -> (130.2197, 22.225)
  line L2745 (130.2197, 22.225) -> (124.7205, 12.7)
  line L2746 (124.7205, 12.7) -> (130.2197, 3.175)
  line L2747 (130.2197, 3.175) -> (141.2182, 3.175)
  line L2748 (146.7175, 12.7) -> (141.2182, 22.225)
  line L2749 (141.2182, 3.175) -> (146.7175, 12.7)
  line L2750 (160.4657, 33.3375) -> (149.4671, 33.3375)
  line L2751 (149.4671, 33.3375) -> (143.9679, 23.8125)
  line L2752 (143.9679, 23.8125) -> (149.4671, 14.2875)
  line L2753 (149.4671, 14.2875) -> (160.4657, 14.2875)
  line L2754 (165.9649, 23.8125) -> (160.4657, 33.3375)
  line L2755 (160.4657, 14.2875) -> (165.9649, 23.8125)
  line L2756 (179.7131, 44.45) -> (168.7145, 44.45)
  line L2757 (168.7145, 44.45) -> (163.2153, 34.925)
  line L2758 (163.2153, 34.925) -> (168.7145, 25.4)
  line L2759 (168.7145, 25.4) -> (179.7131, 25.4)
  line L2760 (185.2123, 34.925) -> (179.7131, 44.45)
  line L2761 (179.7131, 25.4) -> (185.2123, 34.925)
  line L2762 (198.9605, 55.5625) -> (187.962, 55.5625)
  line L2763 (187.962, 55.5625) -> (182.4627, 46.0375)
  line L2764 (182.4627, 46.0375) -> (187.962, 36.5125)
  line L2765 (187.962, 36.5125) -> (198.9605, 36.5125)
  line L2766 (204.4597, 46.0375) -> (198.9605, 55.5625)
  line L2767 (198.9605, 36.5125) -> (204.4597, 46.0375)
  line L2768 (218.2079, 66.675) -> (207.2094, 66.675)
  line L2769 (207.2094, 66.675) -> (201.7101, 57.15)
  line L2770 (201.7101, 57.15) -> (207.2094, 47.625)
  line L2771 (207.2094, 47.625) -> (218.2079, 47.625)
  line L2772 (223.7072, 57.15) -> (218.2079, 66.675)
  line L2773 (218.2079, 47.625) -> (223.7072, 57.15)
  line L2774 (237.4553, 77.7875) -> (226.4568, 77.7875)
  line L2775 (226.4568, 77.7875) -> (220.9575, 68.2625)
  line L2776 (220.9575, 68.2625) -> (226.4568, 58.7375)
  line L2777 (226.4568, 58.7375) -> (237.4553, 58.7375)
  line L2778 (242.9546, 68.2625) -> (237.4553, 77.7875)
  line L2779 (237.4553, 58.7375) -> (242.9546, 68.2625)
  line L2780 (256.7027, 88.9) -> (245.7042, 88.9)
  line L2781 (245.7042, 88.9) -> (240.2049, 79.375)
  line L2782 (240.2049, 79.375) -> (245.7042, 69.85)
  line L2783 (245.7042, 69.85) -> (256.7027, 69.85)
  line L2784 (262.202, 79.375) -> (256.7027, 88.9)
  line L2785 (256.7027, 69.85) -> (262.202, 79.375)
  line L2786 (275.9501, 100.0125) -> (264.9516, 100.0125)
  line L2787 (264.9516, 100.0125) -> (259.4524, 90.4875)
  line L2788 (259.4524, 90.4875) -> (264.9516, 80.9625)
  line L2789 (264.9516, 80.9625) -> (275.9501, 80.9625)
  line L2790 (281.4494, 90.4875) -> (275.9501, 100.0125)
  line L2791 (275.9501, 80.9625) -> (281.4494, 90.4875)
  line L2792 (295.1976, 111.125) -> (284.199, 111.125)
  line L2793 (284.199, 111.125) -> (278.6998, 101.6)
  line L2794 (278.6998, 101.6) -> (284.199, 92.075)
  line L2795 (284.199, 92.075) -> (295.1976, 92.075)
  line L2796 (300.6968, 101.6) -> (295.1976, 111.125)
  line L2797 (295.1976, 92.075) -> (300.6968, 101.6)
  line L2798 (314.445, 122.2375) -> (303.4464, 122.2375)
  line L2799 (303.4464, 122.2375) -> (297.9472, 112.7125)
  line L2800 (297.9472, 112.7125) -> (303.4464, 103.1875)
  line L2801 (303.4464, 103.1875) -> (314.445, 103.1875)
  line L2802 (319.9442, 112.7125) -> (314.445, 122.2375)
  line L2803 (314.445, 103.1875) -> (319.9442, 112.7125)
  line L2804 (333.6924, 133.35) -> (322.6939, 133.35)
  line L2805 (322.6939, 133.35) -> (317.1946, 123.825)
  line L2806 (317.1946, 123.825) -> (322.6939, 114.3)
  line L2807 (322.6939, 114.3) -> (333.6924, 114.3)
  line L2808 (339.1916, 123.825) -> (333.6924, 133.35)
  line L2809 (333.6924, 114.3) -> (339.1916, 123.825)
  line L2810 (352.9398, 144.4625) -> (341.9413, 144.4625)
  line L2811 (341.9413, 144.4625) -> (336.442, 134.9375)
  line L2812 (336.442, 134.9375) -> (341.9413, 125.4125)
  line L2813 (341.9413, 125.4125) -> (352.9398, 125.4125)
  line L2814 (358.4391, 134.9375) -> (352.9398, 144.4625)
  line L2815 (352.9398, 125.4125) -> (358.4391, 134.9375)
  line L2816 (372.1872, 155.575) -> (361.1887, 155.575)
  line L2817 (361.1887, 155.575) -> (355.6894, 146.05)
  line L2818 (355.6894, 146.05) -> (361.1887, 136.525)
  line L2819 (361.1887, 136.525) -> (372.1872, 136.525)
  line L2820 (377.6865, 146.05) -> (372.1872, 155.575)
  line L2821 (372.1872, 136.525) -> (377.6865, 146.05)
  line L2822 (391.4346, 166.6875) -> (380.4361, 166.6875)
  line L2823 (380.4361, 166.6875) -> (374.9368, 157.1625)
  line L2824 (374.9368, 157.1625) -> (380.4361, 147.6375)
  line L2825 (380.4361, 147.6375) -> (391.4346, 147.6375)
  line L2826 (396.9339, 157.1625) -> (391.4346, 166.6875)
  line L2827 (391.4346, 147.6375) -> (396.9339, 157.1625)
  line L2828 (410.682, 177.8) -> (399.6835, 177.8)
  line L2829 (399.6835, 177.8) -> (394.1843, 168.275)
  line L2830 (394.1843, 168.275) -> (399.6835, 158.75)
  line L2831 (399.6835, 158.75) -> (410.682, 158.75)
  line L2832 (416.1813, 168.275) -> (410.682, 177.8)
  line L2833 (410.682, 158.75) -> (416.1813, 168.275)
  line L2834 (429.9295, 188.9125) -> (418.9309, 188.9125)
  line L2835 (418.9309, 188.9125) -> (413.4317, 179.3875)
  line L2836 (413.4317, 179.3875) -> (418.9309, 169.8625)
  line L2837 (418.9309, 169.8625) -> (429.9295, 169.8625)
  line L2838 (435.4287, 179.3875) -> (429.9295, 188.9125)
  line L2839 (429.9295, 169.8625) -> (435.4287, 179.3875)
  line L2840 (449.1769, 200.025) -> (438.1783, 200.025)
  line L2841 (438.1783, 200.025) -> (432.6791, 190.5)
  line L2842 (432.6791, 190.5) -> (438.1783, 180.975)
  line L2843 (438.1783, 180.975) -> (449.1769, 180.975)
  line L2844 (454.6761, 190.5) -> (449.1769, 200.025)
  line L2845 (449.1769, 180.975) -> (454.6761, 190.5)
  line L2846 (468.4243, 211.1375) -> (457.4258, 211.1375)
  line L2847 (457.4258, 211.1375) -> (451.9265, 201.6125)
  line L2848 (451.9265, 201.6125) -> (457.4258, 192.0875)
  line L2849 (457.4258, 192.0875) -> (468.4243, 192.0875)
  line L2850 (473.9235, 201.6125) -> (468.4243, 211.1375)
  line L2851 (468.4243, 192.0875) -> (473.9235, 201.6125)
  line L2852 (487.6717, 222.25) -> (476.6732, 222.25)
  line L2853 (476.6732, 222.25) -> (471.1739, 212.725)
  line L2854 (471.1739, 212.725) -> (476.6732, 203.2)
  line L2855 (476.6732, 203.2) -> (487.6717, 203.2)
  line L2856 (493.171, 212.725) -> (487.6717, 222.25)
  line L2857 (487.6717, 203.2) -> (493.171, 212.725)
  line L2858 (506.9191, 233.3625) -> (495.9206, 233.3625)
  line L2859 (495.9206, 233.3625) -> (490.4213, 223.8375)
  line L2860 (490.4213, 223.8375) -> (495.9206, 214.3125)
  line L2861 (495.9206, 214.3125) -> (506.9191, 214.3125)
  line L2862 (512.4184, 223.8375) -> (506.9191, 233.3625)
  line L2863 (506.9191, 214.3125) -> (512.4184, 223.8375)
  line L2864 (526.1665, 244.475) -> (515.168, 244.475)
  line L2865 (515.168, 244.475) -> (509.6687, 234.95)
  line L2866 (509.6687, 234.95) -> (515.168, 225.425)
  line L2867 (515.168, 225.425) -> (526.1665, 225.425)
  line L2868 (531.6658, 234.95) -> (526.1665, 244.475)
  line L2869 (526.1665, 225.425) -> (531.6658, 234.95)
  line L2870 (545.4139, 255.5875) -> (534.4154, 255.5875)
  line L2871 (534.4154, 255.5875) -> (528.9162, 246.0625)
  line L2872 (528.9162, 246.0625) -> (534.4154, 236.5375)
  line L2873 (534.4154, 236.5375) -> (545.4139, 236.5375)
  line L2874 (550.9132, 246.0625) -> (545.4139, 255.5875)
  line L2875 (545.4139, 236.5375) -> (550.9132, 246.0625)
  line L2876 (564.6614, 266.7) -> (553.6628, 266.7)
  line L2877 (553.6628, 266.7) -> (548.1636, 257.175)
  line L2878 (548.1636, 257.175) -> (553.6628, 247.65)
  line L2879 (553.6628, 247.65) -> (564.6614, 247.65)
  line L2880 (570.1606, 257.175) -> (564.6614, 266.7)
  line L2881 (564.6614, 247.65) -> (570.1606, 257.175)
  line L2882 (583.9088, 277.8125) -> (572.9102, 277.8125)
  line L2883 (572.9102, 277.8125) -> (567.411, 268.2875)
  line L2884 (567.411, 268.2875) -> (572.9102, 258.7625)
  line L2885 (572.9102, 258.7625) -> (583.9088, 258.7625)
  line L2886 (589.408, 268.2875) -> (583.9088, 277.8125)
  line L2887 (583.9088, 258.7625) -> (589.408, 268.2875)
  line L2888 (603.1562, 288.925) -> (592.1577, 288.925)
  line L2889 (592.1577, 288.925) -> (586.6584, 279.4)
  line L2890 (586.6584, 279.4) -> (592.1577, 269.875)
  line L2891 (592.1577, 269.875) -> (603.1562, 269.875)
  line L2892 (608.6554, 279.4) -> (603.1562, 288.925)
  line L2893 (603.1562, 269.875) -> (608.6554, 279.4)
  line L2894 (622.4036, 300.0375) -> (611.4051, 300.0375)
  line L2895 (611.4051, 300.0375) -> (605.9058, 290.5125)
  line L2896 (605.9058, 290.5125) -> (611.4051, 280.9875)
  line L2897 (611.4051, 280.9875) -> (622.4036, 280.9875)
  line L2898 (627.9029, 290.5125) -> (622.4036, 300.0375)
  line L2899 (622.4036, 280.9875) -> (627.9029, 290.5125)
  line L2900 (-532.4413, -344.4875) -> (-543.4398, -344.4875)
  line L2901 (-543.4398, -344.4875) -> (-548.9391, -354.0125)
  line L2902 (-548.9391, -354.0125) -> (-543.4398, -363.5375)
  line L2903 (-543.4398, -363.5375) -> (-532.4413, -363.5375)
  line L2904 (-526.942, -354.0125) -> (-532.4413, -344.4875)
  line L2905 (-532.4413, -363.5375) -> (-526.942, -354.0125)
  line L2906 (-513.1939, -333.375) -> (-524.1924, -333.375)
  line L2907 (-524.1924, -333.375) -> (-529.6916, -342.9)
  line L2908 (-529.6916, -342.9) -> (-524.1924, -352.425)
  line L2909 (-524.1924, -352.425) -> (-513.1939, -352.425)
  line L2910 (-507.6946, -342.9) -> (-513.1939, -333.375)
  line L2911 (-513.1939, -352.425) -> (-507.6946, -342.9)
  line L2912 (-493.9464, -322.2625) -> (-504.945, -322.2625)
  line L2913 (-504.945, -322.2625) -> (-510.4442, -331.7875)
  line L2914 (-510.4442, -331.7875) -> (-504.945, -341.3125)
  line L2915 (-504.945, -341.3125) -> (-493.9464, -341.3125)
  line L2916 (-488.4472, -331.7875) -> (-493.9464, -322.2625)
  line L2917 (-493.9464, -341.3125) -> (-488.4472, -331.7875)
  line L2918 (-474.699, -311.15) -> (-485.6976, -311.15)
  line L2919 (-485.6976, -311.15) -> (-491.1968, -320.675)
  line L2920 (-491.1968, -320.675) -> (-485.6976, -330.2)
  line L2921 (-485.6976, -330.2) -> (-474.699, -330.2)
  line L2922 (-469.1998, -320.675) -> (-474.699, -311.15)
  line L2923 (-474.699, -330.2) -> (-469.1998, -320.675)
  line L2924 (-455.4516, -300.0375) -> (-466.4501, -300.0375)
  line L2925 (-466.4501, -300.0375) -> (-471.9494, -309.5625)
  line L2926 (-471.9494, -309.5625) -> (-466.4501, -319.0875)
  line L2927 (-466.4501, -319.0875) -> (-455.4516, -319.0875)
  line L2928 (-449.9524, -309.5625) -> (-455.4516, -300.0375)
  line L2929 (-455.4516, -319.0875) -> (-449.9524, -309.5625)
  line L2930 (-436.2042, -288.925) -> (-447.2027, -288.925)
  line L2931 (-447.2027, -288.925) -> (-452.702, -298.45)
  line L2932 (-452.702, -298.45) -> (-447.2027, -307.975)
  line L2933 (-447.2027, -307.975) -> (-436.2042, -307.975)
  line L2934 (-430.7049, -298.45) -> (-436.2042, -288.925)
  line L2935 (-436.2042, -307.975) -> (-430.7049, -298.45)
  line L2936 (-416.9568, -277.8125) -> (-427.9553, -277.8125)
  line L2937 (-427.9553, -277.8125) -> (-433.4546, -287.3375)
  line L2938 (-433.4546, -287.3375) -> (-427.9553, -296.8625)
  line L2939 (-427.9553, -296.8625) -> (-416.9568, -296.8625)
  line L2940 (-411.4575, -287.3375) -> (-416.9568, -277.8125)
  line L2941 (-416.9568, -296.8625) -> (-411.4575, -287.3375)
  line L2942 (-397.7094, -266.7) -> (-408.7079, -266.7)
  line L2943 (-408.7079, -266.7) -> (-414.2072, -276.225)
  line L2944 (-414.2072, -276.225) -> (-408.7079, -285.75)
  line L2945 (-408.7079, -285.75) -> (-397.7094, -285.75)
  line L2946 (-392.2101, -276.225) -> (-397.7094, -266.7)
  line L2947 (-397.7094, -285.75) -> (-392.2101, -276.225)
  line L2948 (-378.462, -255.5875) -> (-389.4605, -255.5875)
  line L2949 (-389.4605, -255.5875) -> (-394.9597, -265.1125)
  line L2950 (-394.9597, -265.1125) -> (-389.4605, -274.6375)
  line L2951 (-389.4605, -274.6375) -> (-378.462, -274.6375)
  line L2952 (-372.9627, -265.1125) -> (-378.462, -255.5875)
  line L2953 (-378.462, -274.6375) -> (-372.9627, -265.1125)
  line L2954 (-359.2145, -244.475) -> (-370.2131, -244.475)
  line L2955 (-370.2131, -244.475) -> (-375.7123, -254)
  line L2956 (-375.7123, -254) -> (-370.2131, -263.525)
  line L2957 (-370.2131, -263.525) -> (-359.2145, -263.525)
  line L2958 (-353.7153, -254) -> (-359.2145, -244.475)
  line L2959 (-359.2145, -263.525) -> (-353.7153, -254)
  line L2960 (-339.9671, -233.3625) -> (-350.9657, -233.3625)
  line L2961 (-350.9657, -233.3625) -> (-356.4649, -242.8875)
  line L2962 (-356.4649, -242.8875) -> (-350.9657, -252.4125)
  line L2963 (-350.9657, -252.4125) -> (-339.9671, -252.4125)
  line L2964 (-334.4679, -242.8875) -> (-339.9671, -233.3625)
  line L2965 (-339.9671, -252.4125) -> (-334.4679, -242.8875)
  line L2966 (-320.7197, -222.25) -> (-331.7182, -222.25)
  line L2967 (-331.7182, -222.25) -> (-337.2175, -231.775)
  line L2968 (-337.2175, -231.775) -> (-331.7182, -241.3)
  line L2969 (-331.7182, -241.3) -> (-320.7197, -241.3)
  line L2970 (-315.2205, -231.775) -> (-320.7197, -222.25)
  line L2971 (-320.7197, -241.3) -> (-315.2205, -231.775)
  line L2972 (-301.4723, -211.1375) -> (-312.4708, -211.1375)
  line L2973 (-312.4708, -211.1375) -> (-317.9701, -220.6625)
  line L2974 (-317.9701, -220.6625) -> (-312.4708, -230.1875)
  line L2975 (-312.4708, -230.1875) -> (-301.4723, -230.1875)
  line L2976 (-295.973, -220.6625) -> (-301.4723, -211.1375)
  line L2977 (-301.4723, -230.1875) -> (-295.973, -220.6625)
  line L2978 (-282.2249, -200.025) -> (-293.2234, -200.025)
  line L2979 (-293.2234, -200.025) -> (-298.7227, -209.55)
  line L2980 (-298.7227, -209.55) -> (-293.2234, -219.075)
  line L2981 (-293.2234, -219.075) -> (-282.2249, -219.075)
  line L2982 (-276.7256, -209.55) -> (-282.2249, -200.025)
  line L2983 (-282.2249, -219.075) -> (-276.7256, -209.55)
  line L2984 (-262.9775, -188.9125) -> (-273.976, -188.9125)
  line L2985 (-273.976, -188.9125) -> (-279.4753, -198.4375)
  line L2986 (-279.4753, -198.4375) -> (-273.976, -207.9625)
  line L2987 (-273.976, -207.9625) -> (-262.9775, -207.9625)
  line L2988 (-257.4782, -198.4375) -> (-262.9775, -188.9125)
  line L2989 (-262.9775, -207.9625) -> (-257.4782, -198.4375)
  line L2990 (-243.7301, -177.8) -> (-254.7286, -177.8)
  line L2991 (-254.7286, -177.8) -> (-260.2278, -187.325)
  line L2992 (-260.2278, -187.325) -> (-254.7286, -196.85)
  line L2993 (-254.7286, -196.85) -> (-243.7301, -196.85)
  line L2994 (-238.2308, -187.325) -> (-243.7301, -177.8)
  line L2995 (-243.7301, -196.85) -> (-238.2308, -187.325)
  line L2996 (-224.4826, -166.6875) -> (-235.4812, -166.6875)
  line L2997 (-235.4812, -166.6875) -> (-240.9804, -176.2125)
  line L2998 (-240.9804, -176.2125) -> (-235.4812, -185.7375)
  line L2999 (-235.4812, -185.7375) -> (-224.4826, -185.7375)
  line L3000 (-218.9834, -176.2125) -> (-224.4826, -166.6875)
  line L3001 (-224.4826, -185.7375) -> (-218.9834, -176.2125)
  line L3002 (-205.2352, -155.575) -> (-216.2337, -155.575)
  line L3003 (-216.2337, -155.575) -> (-221.733, -165.1)
  line L3004 (-221.733, -165.1) -> (-216.2337, -174.625)
  line L3005 (-216.2337, -174.625) -> (-205.2352, -174.625)
  line L3006 (-199.736, -165.1) -> (-205.2352, -155.575)
  line L3007 (-205.2352, -174.625) -> (-199.736, -165.1)
  line L3008 (-185.9878, -144.4625) -> (-196.9863, -144.4625)
  line L3009 (-196.9863, -144.4625) -> (-202.4856, -153.9875)